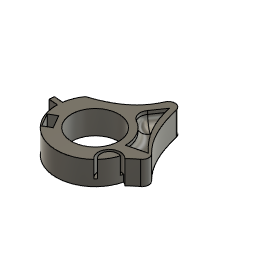
reverseTrigger (Autodesk Fusion 360 design; units mm, degrees)
Autodesk Fusion 360 part; units mm, degrees
sketch "Sketch1" plane through (0, 0, 0) normal (0, 1, 0) x (1, 0, 0)
  circle A0 centre (0, 0) radius 7
  circle A1 centre (0, 0) radius 11.5
  line L0 (-9.4202, 6.5961) -> (5.6542, 28.1247)
  line L1 (0, 11.5) -> (0, -11.5)
  line L2 (-11.5, 0) -> (11.5, 0)
  line L3 (9.9593, 5.75) -> (-9.9593, -5.75)
  line L4 (11.5, 0) -> (17, 0)
  spline S0 degree 5 poles (5.6542, 28.1247) (5.731, 27.3195) (5.897, 25.7291) (6.183, 23.4036) (6.6399, 20.4249) (7.3461, 16.9199) (8.2015, 13.656) (9.2222, 10.6595) (10.4226, 7.9534) (11.8065, 5.5441) (13.3651, 3.4171) (14.7426, 1.9266) (15.8448, 0.9205) (16.6099, 0.2987) (17, 0) knots 0 0 0 0 0 0 0.1 0.2 0.3 0.4 0.5 0.6 0.7 0.8 0.9 1 1 1 1 1 1
  line L5 (0, 0) -> (9.9593, -5.75)
  circle A2 centre (9.9593, -5.75) radius 3.25
  circle A3 centre (9.9593, -5.75) radius 2.5
  line L6 (-6.2362, -6.1986) -> (-8.4862, -2.3014)
  line L7 (-8.4862, -2.3014) -> (-10.6513, -3.5514)
  line L8 (-10.6513, -3.5514) -> (-8.4013, -7.4486)
  line L9 (-8.4013, -7.4486) -> (-6.2362, -6.1986)
  line L10 (-6.2362, -6.1986) -> (-10.6513, -3.5514) construction
  line L11 (-8.4862, -2.3014) -> (-8.4013, -7.4486) construction
  spline S1 degree 5 poles (17, 0) (16.8759, -0.0626) (16.6258, -0.1934) (16.2446, -0.4061) (15.7243, -0.7235) (15.0526, -1.1801) (14.3579, -1.7009) (13.639, -2.2896) (12.8961, -2.9457) (12.1308, -3.6642) (11.3453, -4.4392) (10.7023, -5.1003) (10.2123, -5.6176) (9.8823, -5.972) (9.7165, -6.1515) knots 0 0 0 0 0 0 0.1 0.2 0.3 0.4 0.5 0.6 0.7 0.8 0.9 1 1 1 1 1 1
  point P0 (10, 9)
  point P1 (-15, 0)
  point P2 (-8.4437, -4.875)
  point P3 (14, -2)
  dimension "d1" = 14
  dimension "d2" = 23
  dimension "d6" = 55
  dimension "d39" = 6.5
  dimension "d40" = 5
  dimension "d42" = 4.5
  dimension "d43" = 2.5
  dimension "d44" = 0.5
  dimension "d57" = 30
  dimension "d58" = 30
  constraint coincident A0.centre A1.centre
  constraint vertical L1
  constraint coincident A1 L1.start
  constraint coincident A1 L1.end
  constraint coincident A1 L2.start
  constraint coincident A1 L2.end
  constraint horizontal L2
  constraint coincident A1 L3.start
  constraint coincident A1 L3.end
  constraint parallel L2 L4
  constraint coincident A1 L0.start
  constraint tangent A1 L0
  constraint coincident A0.centre L2
  constraint coincident A0.centre L3
  constraint coincident A1 L5.end
  constraint coincident L5.end A2.centre
  constraint concentric A2 A3
  constraint perpendicular L6 L7
  constraint parallel L6 L8
  constraint parallel L7 L9
  constraint coincident L10 P2
  constraint coincident L11 P2
  constraint coincident L3 P2
  constraint perpendicular L3 L6
  constraint coincident A1 S1.end
  measures "d1" diameter of A0
  measures "d2" diameter of A1
  measures "d6" angle of L0 L4
  measures "d39" diameter of A2
  measures "d40" diameter of A3
  measures "d42" distance of L7.end L8.end
  measures "d43" distance of L6.end L7.end
  measures "d44" distance of L3.end L8
  measures "d57" angle of L2 L5
  measures "d58" angle of L2 L3
extrude "Extrude1" add sketch "Sketch1" along normal blind 7 contours A0 A1 L2 L5 A2 | A0 A1 L2 L3 | A0 A1 L1 L3 | A0 A1 L1 L5 A2 | A1 L4 A2 S1 | A1 L0 L4 S0 | A0 A1 L1 L2 | A0 A1 L1 L3 L6 L8 L9 | A0 A1 L2 L3 L6 L7 L8 | A1 L5 A3 | A1 L5 A3 makes body 1 at (-1.7746, 0, -13.8484) makes body 2 at (10.1431, 4.6667, 3.2568)
sketch "Sketch6" plane through (0, 0, 0) normal (0, -1, 0) x (1, 0, 0)
  arc A0 (7.9529, 8.3067) -> (-9.4202, -6.5961) centre (0, 0) ccw
  line L0 (-9.4202, -6.5961) -> (5.6542, -28.1247)
  spline S0 degree 5 poles (5.6542, -28.1247) (5.731, -27.3195) (5.897, -25.7291) (6.183, -23.4036) (6.6399, -20.4249) (7.3461, -16.9199) (8.2015, -13.656) (9.2222, -10.6595) (10.4226, -7.9534) (11.8065, -5.5441) (13.3651, -3.4171) (14.7426, -1.9266) (15.8448, -0.9205) (16.6099, -0.2987) (17, 0) knots 0 0 0 0 0 0 0.1 0.2 0.3 0.4 0.5 0.6 0.7 0.8 0.9 1 1 1 1 1 1
  circle A1 centre (0, 0) radius 11.5
  spline S1 degree 5 poles (17, 0) (16.8759, 0.0626) (16.6258, 0.1934) (16.2446, 0.4061) (15.7243, 0.7235) (15.0526, 1.1801) (14.3579, 1.7009) (13.673, 2.2618) (13.1147, 2.7527) (12.6962, 3.1372) (12.4258, 3.3918) (12.3081, 3.5038) knots 0 0 0 0 0 0 0.1 0.2 0.3 0.4 0.5 0.6 0.676399 0.676399 0.676399 0.676399 0.676399 0.676399
  line L1 (-8.4013, 7.4486) -> (-6.2362, 6.1986)
  line L2 (-6.2362, 6.1986) -> (-8.4862, 2.3014)
  line L3 (-8.4862, 2.3014) -> (-10.6513, 3.5514)
  line L4 (-10.6513, 3.5514) -> (-8.4013, 7.4486)
  arc A2 (7.9529, 8.3067) -> (12.3081, 3.5038) centre (9.9593, 5.75) ccw
  arc A3 (10.9666, 3.4619) -> (8.4814, 7.7664) centre (0, 0) ccw
  line L5 (19.0486, 0.0972) -> (12.3081, 3.5038)
  circle A4 centre (0, 0) radius 7
  arc A5 (8.4814, 7.7664) -> (10.9666, 3.4619) centre (9.9593, 5.75) ccw
  constraint coincident S1.end A2.end
extrude "Extrude6" add sketch "Sketch6" against normal blind 2 contours A1 A2 A5 | L0 S0 A1 S1 A2 | A1 A3 A5 | L1 L2 L3 L4 bodies 2 1
sketch "Sketch3" plane through (0, 7, 0) normal (0, 1, 0) x (-1, 0, 0)
  line L0 (-5.6542, -28.1247) -> (9.4202, -6.5961)
  arc A0 (9.4202, -6.5961) -> (-7.9529, 8.3067) centre (0, 0) ccw
  spline S0 degree 5 poles (-17, 0) (-16.6099, -0.2987) (-15.8448, -0.9205) (-14.7426, -1.9266) (-13.3651, -3.4171) (-11.8065, -5.5441) (-10.4226, -7.9534) (-9.2222, -10.6595) (-8.2015, -13.656) (-7.3461, -16.9199) (-6.6399, -20.4249) (-6.183, -23.4036) (-5.897, -25.7291) (-5.731, -27.3195) (-5.6542, -28.1247) knots -1 -1 -1 -1 -1 -1 -0.9 -0.8 -0.7 -0.6 -0.5 -0.4 -0.3 -0.2 -0.1 0 0 0 0 0 0
  circle A1 centre (0, 0) radius 9
  line L1 (-1.0551, -8.9379) -> (-6, -16)
  line L2 (7.3724, -5.1622) -> (9.4202, -6.5961)
  line L3 (-14.3844, -1.3743) -> (-9, 0)
  spline S1 degree 5 poles (-12.3081, 3.5038) (-12.4258, 3.3918) (-12.6962, 3.1372) (-13.1147, 2.7527) (-13.673, 2.2618) (-14.3579, 1.7009) (-15.0526, 1.1801) (-15.7243, 0.7235) (-16.2446, 0.4061) (-16.6258, 0.1934) (-16.8759, 0.0626) (-17, 0) knots -0.676399 -0.676399 -0.676399 -0.676399 -0.676399 -0.676399 -0.6 -0.5 -0.4 -0.3 -0.2 -0.1 0 0 0 0 0 0
  spline S2 degree 5 poles (-6, -16) (-6.0772, -15.6555) (-6.2395, -14.9709) (-6.5067, -13.9578) (-6.9112, -12.6346) (-7.5025, -11.0299) (-8.1873, -9.4789) (-8.9731, -7.9861) (-9.8641, -6.5538) (-10.8562, -5.1796) (-11.9418, -3.8591) (-12.8789, -2.8422) (-13.6178, -2.1003) (-14.1263, -1.6148) (-14.3844, -1.3743) knots 0 0 0 0 0 0 0.1 0.2 0.3 0.4 0.5 0.6 0.7 0.8 0.9 1 1 1 1 1 1
  line L4 (6.2362, 6.1986) -> (8.4013, 7.4486)
  line L5 (8.4013, 7.4486) -> (10.6513, 3.5514)
  line L6 (10.6513, 3.5514) -> (8.4862, 2.3014)
  line L7 (8.4862, 2.3014) -> (6.2362, 6.1986)
  arc A2 (-12.3081, 3.5038) -> (-7.9529, 8.3067) centre (-9.9593, 5.75) ccw
  circle A3 centre (0, 0) radius 7
  point P0 (-9, -8)
  dimension "d19" = 18
  constraint concentric A0 A1
  constraint coincident L0.end A0.start
  constraint coincident A1 L2.start
  constraint coincident A1 L1.start
  constraint parallel L0 L1
  constraint perpendicular L1 L2
  constraint coincident A1 L3.end
  constraint coincident L1 S2.start
  measures "d19" diameter of A1
extrude "Extrude3" cut sketch "Sketch3" against normal blind 4 contours A1 L1 L3 S2 bodies 2
fillet "Fillet2" radius 3 4 edges at (1.0551, 5, -8.9379) (3.5275, 3, -12.469) (11.6922, 3, -0.6871) (6.7267, 3, -5.9793) on bodies 2
sketch "Sketch5" plane through (0, 3, 0) normal (0, 1, 0) x (-1, 0, 0)
  line L0 (7.0967, 0.1053) -> (6.9709, -1.3346)
  line L1 (6.9709, -1.3346) -> (14.0047, -1.9492)
  line L2 (14.0047, -1.9492) -> (14.1305, -0.5094)
  line L3 (14.1305, -0.5094) -> (7.0967, 0.1053)
  line L4 (0, 0) -> (14.0676, -1.2293)
  line L5 (0, -18) -> (0, 20)
  spline S0 degree 5 poles (-7.0585, -12.2813) (-7.1466, -12.0306) (-7.3544, -11.4599) (-7.7014, -10.5801) (-8.1025, -9.6811) (-8.5462, -8.8066) (-8.8951, -8.1789) (-9.0868, -7.8497) (-9.1089, -7.812) knots 0.22252 0.22252 0.22252 0.22252 0.22252 0.22252 0.3 0.4 0.5 0.51297 0.51297 0.51297 0.51297 0.51297 0.51297
  line L6 (-7.0585, -12.2813) -> (-5.8107, -10.4993)
  arc A0 (-9.1089, -7.812) -> (-5.8107, -10.4993) centre (0, 0) ccw
  constraint perpendicular L0 L1
  constraint parallel L0 L2
  constraint parallel L1 L3
  constraint coincident A0.centre L4
  constraint vertical L5
  constraint coincident L4.start L5
  constraint midpoint L2 L4.end
  constraint midpoint L0 L4
  constraint coincident L4.start A0.centre
extrude "Extrude5" add sketch "Sketch5" along normal blind 4 and the other way blind 1 contours L0 L2 L3 L4 | L0 L1 L2 L4 bodies 2
sketch "Sketch8" plane through (0, 7, 0) normal (0, 1, 0) x (-1, 0, 0)
  spline S0 degree 5 poles (-17, 0) (-16.6099, -0.2987) (-15.8448, -0.9205) (-14.7426, -1.9266) (-13.3651, -3.4171) (-11.8065, -5.5441) (-10.4226, -7.9534) (-9.2222, -10.6595) (-8.2015, -13.656) (-7.3461, -16.9199) (-6.6399, -20.4249) (-6.183, -23.4036) (-5.897, -25.7291) (-5.731, -27.3195) (-5.6542, -28.1247) knots -1 -1 -1 -1 -1 -1 -0.9 -0.8 -0.7 -0.6 -0.5 -0.4 -0.3 -0.2 -0.1 0 0 0 0 0 0
  line L0 (-5.6542, -28.1247) -> (9.4202, -6.5961)
  arc A0 (11.4966, -0.2792) -> (-7.9529, 8.3067) centre (0, 0) ccw
  line L1 (14.0047, -1.9492) -> (14.1305, -0.5094)
  line L2 (14.1305, -0.5094) -> (11.4966, -0.2792)
  arc A1 (-9, 0) -> (-4.358, -7.8745) centre (0, 0) ccw
  line L3 (-3.3532, -12.22) -> (-6, -16)
  line L4 (-14.3844, -1.3743) -> (-9, 0)
  spline S1 degree 5 poles (-6, -16) (-6.0772, -15.6555) (-6.2395, -14.9709) (-6.5067, -13.9578) (-6.9112, -12.6346) (-7.5025, -11.0299) (-8.1873, -9.4789) (-8.9731, -7.9861) (-9.8641, -6.5538) (-10.8562, -5.1796) (-11.9418, -3.8591) (-12.8789, -2.8422) (-13.6178, -2.1003) (-14.1263, -1.6148) (-14.3844, -1.3743) knots 0 0 0 0 0 0 0.1 0.2 0.3 0.4 0.5 0.6 0.7 0.8 0.9 1 1 1 1 1 1
  spline S2 degree 5 poles (-12.3081, 3.5038) (-12.4258, 3.3918) (-12.6962, 3.1372) (-13.1147, 2.7527) (-13.673, 2.2618) (-14.3579, 1.7009) (-15.0526, 1.1801) (-15.7243, 0.7235) (-16.2446, 0.4061) (-16.6258, 0.1934) (-16.8759, 0.0626) (-17, 0) knots -0.676399 -0.676399 -0.676399 -0.676399 -0.676399 -0.676399 -0.6 -0.5 -0.4 -0.3 -0.2 -0.1 0 0 0 0 0 0
  line L5 (6.2362, 6.1986) -> (8.4013, 7.4486)
  line L6 (8.4013, 7.4486) -> (10.6513, 3.5514)
  line L7 (10.6513, 3.5514) -> (8.4862, 2.3014)
  line L8 (8.4862, 2.3014) -> (6.2362, 6.1986)
  arc A2 (-12.3081, 3.5038) -> (-7.9529, 8.3067) centre (-9.9593, 5.75) ccw
  line L9 (11.3708, -1.719) -> (14.0047, -1.9492)
  arc A3 (-3.3532, -12.22) -> (-4.358, -7.8745) centre (-5.8107, -10.4993) ccw
  arc A4 (9.4202, -6.5961) -> (11.3708, -1.719) centre (0, 0) ccw
  circle A5 centre (0, 0) radius 7
sketch "Sketch9" plane through (0, 7, 0) normal (0, 1, 0) x (-1, 0, 0)
  arc A0 (11.4966, -0.2792) -> (-7.9529, 8.3067) centre (0, 0) ccw
  arc A1 (-12.3081, 3.5038) -> (-7.9529, 8.3067) centre (-9.9593, 5.75) ccw
  spline S0 degree 5 poles (-12.3081, 3.5038) (-12.4258, 3.3918) (-12.6962, 3.1372) (-13.1147, 2.7527) (-13.673, 2.2618) (-14.3579, 1.7009) (-15.0526, 1.1801) (-15.7243, 0.7235) (-16.2446, 0.4061) (-16.6258, 0.1934) (-16.8759, 0.0626) (-17, 0) knots -0.676399 -0.676399 -0.676399 -0.676399 -0.676399 -0.676399 -0.6 -0.5 -0.4 -0.3 -0.2 -0.1 0 0 0 0 0 0
  spline S1 degree 5 poles (-17, 0) (-16.6099, -0.2987) (-15.8448, -0.9205) (-14.7426, -1.9266) (-13.3651, -3.4171) (-11.8065, -5.5441) (-10.4226, -7.9534) (-9.2222, -10.6595) (-8.2015, -13.656) (-7.3461, -16.9199) (-6.6399, -20.4249) (-6.183, -23.4036) (-5.897, -25.7291) (-5.731, -27.3195) (-5.6542, -28.1247) knots -1 -1 -1 -1 -1 -1 -0.9 -0.8 -0.7 -0.6 -0.5 -0.4 -0.3 -0.2 -0.1 0 0 0 0 0 0
  line L0 (-5.6542, -28.1247) -> (9.4202, -6.5961)
  arc A2 (9.4202, -6.5961) -> (11.3708, -1.719) centre (0, 0) ccw
  line L1 (11.3708, -1.719) -> (14.0047, -1.9492)
  line L2 (14.0047, -1.9492) -> (14.1305, -0.5094)
  line L3 (14.1305, -0.5094) -> (11.4966, -0.2792)
  arc A3 (-9, 0) -> (-4.358, -7.8745) centre (0, 0) ccw
  arc A4 (-3.3532, -12.22) -> (-4.358, -7.8745) centre (-5.8107, -10.4993) ccw
  line L4 (-3.3532, -12.22) -> (-6, -16)
  spline S2 degree 5 poles (-6, -16) (-6.0772, -15.6555) (-6.2395, -14.9709) (-6.5067, -13.9578) (-6.9112, -12.6346) (-7.5025, -11.0299) (-8.1873, -9.4789) (-8.9731, -7.9861) (-9.8641, -6.5538) (-10.8562, -5.1796) (-11.9418, -3.8591) (-12.8789, -2.8422) (-13.6178, -2.1003) (-14.1263, -1.6148) (-14.3844, -1.3743) knots 0 0 0 0 0 0 0.1 0.2 0.3 0.4 0.5 0.6 0.7 0.8 0.9 1 1 1 1 1 1
  line L5 (-14.3844, -1.3743) -> (-9, 0)
  line L6 (6.2362, 6.1986) -> (8.4013, 7.4486)
  line L7 (8.4013, 7.4486) -> (10.6513, 3.5514)
  line L8 (10.6513, 3.5514) -> (8.4862, 2.3014)
  line L9 (8.4862, 2.3014) -> (6.2362, 6.1986)
  circle A5 centre (0, 0) radius 7
  spline S3 degree 5 poles (9.4202, -6.5961) (8.8133, -6.7836) (7.6264, -7.18) (5.9266, -7.8388) (3.8241, -8.8475) (1.4875, -10.3405) (-0.5322, -12.0857) (-2.2102, -14.1028) (-3.535, -16.4011) (-4.5228, -18.9675) (-5.2, -21.781) (-5.5142, -24.213) (-5.63, -26.1324) (-5.6549, -27.4536) (-5.6542, -28.1247) knots 0 0 0 0 0 0 0.1 0.2 0.3 0.4 0.5 0.6 0.7 0.8 0.9 1 1 1 1 1 1
  point P0 (-2, -14)
  constraint coincident L0.end A2.start
  constraint coincident S1.end L0.start
extrude "Extrude8" cut sketch "Sketch9" against normal blind 10 contours L0 S3 bodies 2
fillet "Fillet7" radius 2 2 edges at (17, 3.5, 0) (5.6542, 3.5, -28.1247) on bodies 2
